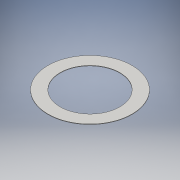
# Autodesk Inventor part: Arruela da chave seletora
Saved by Autodesk Inventor 2016 (Build 200138000, 138)
## iProperties
Created: 2018-11-13
Part Number: Arruela da chave seletora
Material: Genérico
Document SubType Name: Modeling
Designer: thiag
Density: 1 g/cm^3
Appearance: Padrão
Author: thiag
Autodesk Inventor part; units mm, degrees
ref_plane "YZ Plane" through (0, 0, 0) normal (1, 0, 0) x (0, 1, 0)
ref_plane "XZ Plane" through (0, 0, 0) normal (0, 1, 0) x (-1, 0, 0)
ref_plane "XY Plane" through (0, 0, 0) normal (0, 0, 1) x (1, 0, 0)
sketch "Esboço1" plane through (0, 0, 0) normal (0, 0, 1) x (1, 0, 0)
  circle A0 centre (0, 0) radius 8.95
  circle A1 centre (0, 0) radius 6.35
  constraints: 2 centre point, 2 coincident
extrude "Extrusão1" add sketch "Esboço1" along normal blind 0.1
